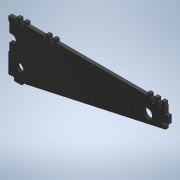
# Autodesk Inventor part: 10_ramie
Saved by Autodesk Inventor 2020.2 (Build 242310000, 310)
## iProperties
Created: 2017-10-07
Part Number: 10_ramie
Material: Ogólny
Document SubType Name: Modeling
Designer: Haras2
Density: 1 g/cm^3
Appearance: Gładki - czarny
Mass: 330.705 g
Surface Area: 962.933 cm^2
Volume: 330.705 cm^3
Author: Haras2
Autodesk Inventor part; units mm, degrees
ref_plane "YZ Plane" through (0, 0, 0) normal (1, 0, 0) x (0, 1, 0)
ref_plane "XZ Plane" through (0, 0, 0) normal (0, 1, 0) x (-1, 0, 0)
ref_plane "XY Plane" through (0, 0, 0) normal (0, 0, 1) x (1, 0, 0)
sketch "Szkic1" plane through (0, 0, 0) normal (0, 1, 0) x (-1, 0, 0)
  line L0 (0, 0) -> (0, -12)
  line L1 (0, -12) -> (-3, -15)
  line L2 (0, -137) -> (-15.5, -137)
  line L3 (-15.5, -137) -> (-15.5, -145)
  line L4 (-15.5, -145) -> (-35.5, -145)
  line L5 (-35.5, -145) -> (-35.5, -137)
  line L6 (-35.5, -137) -> (-47.5, -137)
  line L7 (-47.5, -137) -> (-421.5, -55)
  line L8 (-421.5, -55) -> (-421.5, -39.5)
  line L9 (-421.5, -39.5) -> (-429.5, -39.5)
  line L10 (-429.5, -39.5) -> (-429.5, -19.5)
  line L11 (-429.5, -19.5) -> (-421.5, -19.5)
  line L12 (-421.5, -19.5) -> (-421.5, 0)
  line L13 (-421.5, 0) -> (-419.5, 0)
  line L14 (-419.5, 0) -> (-419.5, 8)
  line L15 (-419.5, 8) -> (-411.5, 8)
  line L16 (-411.5, 8) -> (-411.5, 0)
  line L17 (-411.5, 0) -> (-400.5, 0)
  line L18 (-400.5, 0) -> (-400.5, 8)
  line L19 (-400.5, 8) -> (-392.5, 8)
  line L20 (-392.5, 8) -> (-392.5, 0)
  line L21 (-392.5, 0) -> (-381.5, 0)
  line L22 (-381.5, 0) -> (-381.5, 8)
  line L23 (-381.5, 8) -> (-373.5, 8)
  line L24 (-373.5, 8) -> (-373.5, 0)
  line L25 (-373.5, 0) -> (-128.5, 0)
  line L26 (-128.5, 0) -> (-128.5, 8)
  line L27 (-128.5, 8) -> (-120.5, 8)
  line L28 (-120.5, 8) -> (-120.5, 0)
  line L29 (-120.5, 0) -> (-110, 0)
  line L30 (-110, 0) -> (-110, 8)
  line L31 (-110, 8) -> (-102, 8)
  line L32 (-102, 8) -> (-102, 0)
  line L33 (-102, 0) -> (-50, 0)
  line L34 (-50, 0) -> (-50, 8)
  line L35 (-50, 8) -> (-42, 8)
  line L36 (-42, 8) -> (-42, 0)
  line L37 (-42, 0) -> (-31.5, 0)
  line L38 (-31.5, 0) -> (-31.5, 8)
  line L39 (-31.5, 8) -> (-23.5, 8)
  line L40 (-23.5, 8) -> (-23.5, 0)
  line L41 (-23.5, 0) -> (0, 0)
  line L42 (0, -137) -> (0, -84)
  line L43 (0, -84) -> (-3, -81)
  line L44 (-3, -49.75) -> (-9.75, -49.75) construction
  line L45 (-3, -60) -> (-9.75, -60)
  line L46 (-9.75, -39.5) -> (-3, -39.5)
  arc A0 (-9.75, -39.5) -> (-9.75, -60) centre (-9.75, -49.75) ccw
  line L47 (-3, -81) -> (-3, -60)
  line L48 (-3, -39.5) -> (-3, -15)
  line L49 (-385.25, -7) -> (-384, -7)
  line L50 (-384, -7) -> (-384, -4)
  line L51 (-384, -4) -> (-385.25, -4)
  line L52 (-385.25, -4) -> (-385.25, 0)
  line L53 (-385.25, 0) -> (-388.75, 0)
  line L54 (-388.75, 0) -> (-388.75, -4)
  line L55 (-388.75, -4) -> (-390, -4)
  line L56 (-390, -4) -> (-390, -7)
  line L57 (-390, -7) -> (-388.75, -7)
  line L58 (-388.75, -7) -> (-388.75, -12)
  line L59 (-388.75, -12) -> (-385.25, -12)
  line L60 (-385.25, -12) -> (-385.25, -7)
  line L61 (-387, 0) -> (-387, -12) construction
  line L62 (-404.25, -7) -> (-403, -7)
  line L63 (-403, -7) -> (-403, -4)
  line L64 (-403, -4) -> (-404.25, -4)
  line L65 (-404.25, -4) -> (-404.25, 0)
  line L66 (-404.25, 0) -> (-407.75, 0)
  line L67 (-407.75, 0) -> (-407.75, -4)
  line L68 (-407.75, -4) -> (-409, -4)
  line L69 (-409, -4) -> (-409, -7)
  line L70 (-409, -7) -> (-407.75, -7)
  line L71 (-407.75, -7) -> (-407.75, -12)
  line L72 (-407.75, -12) -> (-404.25, -12)
  line L73 (-404.25, -12) -> (-404.25, -7)
  line L74 (-406, 0) -> (-406, -12) construction
  line L75 (-414.5, -43.5) -> (-414.5, -42.25)
  line L76 (-414.5, -42.25) -> (-417.5, -42.25)
  line L77 (-417.5, -42.25) -> (-417.5, -43.5)
  line L78 (-417.5, -43.5) -> (-421.5, -43.5)
  line L79 (-421.5, -43.5) -> (-421.5, -47)
  line L80 (-421.5, -47) -> (-417.5, -47)
  line L81 (-417.5, -47) -> (-417.5, -48.25)
  line L82 (-417.5, -48.25) -> (-414.5, -48.25)
  line L83 (-414.5, -48.25) -> (-414.5, -47)
  line L84 (-414.5, -47) -> (-409.5, -47)
  line L85 (-409.5, -47) -> (-409.5, -43.5)
  line L86 (-409.5, -43.5) -> (-414.5, -43.5)
  line L87 (-421.5, -45.25) -> (-409.5, -45.25) construction
  line L88 (-113.5, -7) -> (-112.25, -7)
  line L89 (-112.25, -7) -> (-112.25, -4)
  line L90 (-112.25, -4) -> (-113.5, -4)
  line L91 (-113.5, -4) -> (-113.5, 0)
  line L92 (-113.5, 0) -> (-117, 0)
  line L93 (-117, 0) -> (-117, -4)
  line L94 (-117, -4) -> (-118.25, -4)
  line L95 (-118.25, -4) -> (-118.25, -7)
  line L96 (-118.25, -7) -> (-117, -7)
  line L97 (-117, -7) -> (-117, -12)
  line L98 (-117, -12) -> (-113.5, -12)
  line L99 (-113.5, -12) -> (-113.5, -7)
  line L100 (-115.25, 0) -> (-115.25, -12) construction
  line L101 (-95, -7) -> (-93.75, -7)
  line L102 (-93.75, -7) -> (-93.75, -4)
  line L103 (-93.75, -4) -> (-95, -4)
  line L104 (-95, -4) -> (-95, 0)
  line L105 (-95, 0) -> (-98.5, 0)
  line L106 (-98.5, 0) -> (-98.5, -4)
  line L107 (-98.5, -4) -> (-99.75, -4)
  line L108 (-99.75, -4) -> (-99.75, -7)
  line L109 (-99.75, -7) -> (-98.5, -7)
  line L110 (-98.5, -7) -> (-98.5, -12)
  line L111 (-98.5, -12) -> (-95, -12)
  line L112 (-95, -12) -> (-95, -7)
  line L113 (-96.75, 0) -> (-96.75, -12) construction
  line L114 (-35, -7) -> (-33.75, -7)
  line L115 (-33.75, -7) -> (-33.75, -4)
  line L116 (-33.75, -4) -> (-35, -4)
  line L117 (-35, -4) -> (-35, 0)
  line L118 (-35, 0) -> (-38.5, 0)
  line L119 (-38.5, 0) -> (-38.5, -4)
  line L120 (-38.5, -4) -> (-39.75, -4)
  line L121 (-39.75, -4) -> (-39.75, -7)
  line L122 (-39.75, -7) -> (-38.5, -7)
  line L123 (-38.5, -7) -> (-38.5, -12)
  line L124 (-38.5, -12) -> (-35, -12)
  line L125 (-35, -12) -> (-35, -7)
  line L126 (-36.75, 0) -> (-36.75, -12) construction
  line L127 (-16.5, -7) -> (-15.25, -7)
  line L128 (-15.25, -7) -> (-15.25, -4)
  line L129 (-15.25, -4) -> (-16.5, -4)
  line L130 (-16.5, -4) -> (-16.5, 0)
  line L131 (-16.5, 0) -> (-20, 0)
  line L132 (-20, 0) -> (-20, -4)
  line L133 (-20, -4) -> (-21.25, -4)
  line L134 (-21.25, -4) -> (-21.25, -7)
  line L135 (-21.25, -7) -> (-20, -7)
  line L136 (-20, -7) -> (-20, -12)
  line L137 (-20, -12) -> (-16.5, -12)
  line L138 (-16.5, -12) -> (-16.5, -7)
  line L139 (-18.25, 0) -> (-18.25, -12) construction
  line L140 (-11.75, -130) -> (-13, -130)
  line L141 (-13, -130) -> (-13, -133)
  line L142 (-13, -133) -> (-11.75, -133)
  line L143 (-11.75, -133) -> (-11.75, -137)
  line L144 (-11.75, -137) -> (-8.25, -137)
  line L145 (-8.25, -137) -> (-8.25, -133)
  line L146 (-8.25, -133) -> (-7, -133)
  line L147 (-7, -133) -> (-7, -130)
  line L148 (-7, -130) -> (-8.25, -130)
  line L149 (-8.25, -130) -> (-8.25, -125)
  line L150 (-8.25, -125) -> (-11.75, -125)
  line L151 (-11.75, -125) -> (-11.75, -130)
  line L152 (-10, -137) -> (-10, -125) construction
  line L153 (-42.75, -130) -> (-44, -130)
  line L154 (-44, -130) -> (-44, -133)
  line L155 (-44, -133) -> (-42.75, -133)
  line L156 (-42.75, -133) -> (-42.75, -137)
  line L157 (-42.75, -137) -> (-39.25, -137)
  line L158 (-39.25, -137) -> (-39.25, -133)
  line L159 (-39.25, -133) -> (-38, -133)
  line L160 (-38, -133) -> (-38, -130)
  line L161 (-38, -130) -> (-39.25, -130)
  line L162 (-39.25, -130) -> (-39.25, -125)
  line L163 (-39.25, -125) -> (-42.75, -125)
  line L164 (-42.75, -125) -> (-42.75, -130)
  line L165 (-41, -137) -> (-41, -125) construction
  point P0 (0, 0)
  point P1 (-30, -107)
  dimension "d5" = 137
  dimension "d6" = 45
  dimension "d7" = 12
  dimension "d8" = 53
  dimension "d9" = 23.5
  dimension "d10" = 8
  dimension "d11" = 10.5
  dimension "d12" = 8
  dimension "d13" = 10.5
  dimension "d14" = 11
  dimension "d15" = 11
  dimension "d16" = 421.5
  dimension "d17" = 55
  dimension "d18" = 8
  dimension "d19" = 20
  dimension "d20" = 19.5
  dimension "d21" = 102
  dimension "d22" = 373.5
  dimension "d23" = 20
  dimension "d24" = 15.5
  dimension "d25" = 8
  dimension "d26" = 47.5
  dimension "d27" = 3
  dimension "d28" = 20.5
  dimension "d29" = 39.5
  dimension "d30" = 17
  dimension "d31" = 4
  dimension "d32" = 3.5
  dimension "d33" = 3.5
  dimension "d34" = 3.75
  dimension "d35" = 3.75
  dimension "d38" = 30
  dimension "d39" = 30
  constraints: 99 end point, 30 point on line, 26 perpendicular, 16 horizontal, 8 collinear, 6 vertical, 2 parallel, 2 point on circle, 2 tangent, 1 centre point, 1 coincident
  measures "d5" distance between parallel lines of L2 L41
  measures "d6" angle of L0 L1
  measures "d7" distance of L0.start L0.end
  measures "d8" distance of L2.start L43.start
  measures "d9" distance between parallel lines of L0 L40
  measures "d10" distance of L38.end L39.end
  measures "d11" distance between parallel lines of L36 L38
  measures "d12" distance of L39.end L40.end
  measures "d13" distance between parallel lines of L28 L30
  measures "d14" distance between parallel lines of L20 L22
  measures "d15" distance between parallel lines of L16 L18
  measures "d16" distance between parallel lines of L0 L12
  measures "d17" distance from line of L13 L8.start
  measures "d18" distance of L11.start L12.start
  measures "d19" distance of L10.start L11.start
  measures "d20" distance between parallel lines of L13 L11
  measures "d21" distance between parallel lines of L0 L32
  measures "d22" distance between parallel lines of L0 L24
  measures "d23" distance of L3.end L4.end
  measures "d24" distance between parallel lines of L42 L3
  measures "d25" distance of L3.start L3.end
  measures "d26" distance from line of L6.end L42
  measures "d27" distance between parallel lines of L0 L48
  measures "d28" distance between parallel lines of L45 L46
  measures "d29" distance between parallel lines of L41 L46
  measures "d38" distance from line of L42 point (-30, -107)
  measures "d39" distance from line of L2 point (-30, -107)
extrude "Wyciągnięcie proste1" add sketch "Szkic1" along normal blind 8 contours L0 L1 L48 L46 A0 L45 L47 L43 L42 L2 L145 L146 L147 L148 L149 L150 L151 L140 L141 L142 L143 L3 L4 L5 L6 L158 L159 L160 L161 L162 L163 L164 L153 L154 L155 L156 L7 L8 L80 L81 L82 L83 L84 L85 L86 L75 L76 L77 L78 L9 L10 L11 L12 L13 L14 L15 L16 L17 L67 L68 L69 L70 L71 L72 L73 L62 L63 L64 L65 L18 L19 L20 L21 L54 L55 L56 L57 L58 L59 L60 L49 L50 L51 L52 L22 L23 L24 L25 L26 L27 L28 L29 L93 L94 L95 L96 L97 L98 L99 L88 L89 L90 L91 L30 L31 L32 L33 L106 L107 L108 L109 L110 L111 L112 L101 L102 L103 L104 L34 L35 L36 L37 L119 L120 L121 L122 L123 L124 L125 L114 L115 L116 L117 L38 L39 L40 L41 L132 L133 L134 L135 L136 L137 L138 L127 L128 L129 L130
sketch "Szkic2" plane through (0, 8, 0) normal (0, 1, 0) x (1, 0, 0)
  line L0 (0, 12) -> (0, 0) projected
  line L1 (50, 0) -> (95, 0) projected
  line L2 (0, 137) -> (0, 84) projected
  line L3 (8.25, 137) -> (0, 137) projected
  line L4 (128.5, 0) -> (373.5, 0) projected
  point P0 (30, 107)
  point P1 (131.5, 6)
  point P2 (131.5, 92.75)
  point P3 (80, 85)
  point P4 (80, 35)
  point P5 (223, 6)
  point P6 (230, 35)
  point P7 (223, 92)
  point P8 (373.5, 42)
  point P9 (338, 46.75)
  dimension "d56" = 80
  dimension "d57" = 35
  dimension "d58" = 30
  dimension "d59" = 30
  dimension "d63" = 92.75
  dimension "d64" = 6
  dimension "d65" = 131.5
  dimension "d66" = 92
  dimension "d67" = 223
  dimension "d69" = 46.75
  dimension "d70" = 42
  dimension "d71" = 373.5
  dimension "d72" = 338
  dimension "d95" = 50
  dimension "d96" = 150
  constraints: 3 vertical alignment, 2 horizontal alignment
  measures "d56" distance from line of L0 point (80, 35)
  measures "d57" distance from line of L1 point (80, 35)
  measures "d58" distance from line of L2 point (30, 107)
  measures "d59" distance from line of point (30, 107) L3
  measures "d63" distance from line of L1 point (131.5, 92.75)
  measures "d64" distance from line of L1 point (131.5, 6)
  measures "d65" distance from line of point (131.5, 6) L0
  measures "d66" distance from line of L4 point (223, 92)
  measures "d67" distance from line of L2 point (223, 92)
  measures "d69" distance from line of L4 point (338, 46.75)
  measures "d70" distance from line of L4 point (373.5, 42)
  measures "d71" distance from line of L0 point (373.5, 42)
  measures "d72" distance from line of point (338, 46.75) L0
  measures "d95" distance of point (80, 85) point (80, 35)
  measures "d96" distance of point (230, 35) point (80, 35)
hole "Otwór1" at (30, 8, -107) at (131.5, 8, -6) at (131.5, 8, -92.75) at (80, 8, -85) at (80, 8, -35) at (223, 8, -6) at (230, 8, -35) at (223, 8, -92) at (373.5, 8, -42) at (338, 8, -46.75) direction (0, -1, 0) diameter 3.5 end through all
sketch "Szkic3" plane through (0, 8, 0) normal (0, 1, 0) x (1, 0, 0)
  circle A0 centre (30, 107) radius 1.75 projected
  point P0 (0, 0)
  constraints: 1 coincident
hole "Otwór2" at (30, 8, -107) direction (0, -1, 0) diameter 20 end through all
sketch "Szkic4" plane through (0, 8, 0) normal (0, 1, 0) x (1, 0, 0)
  circle A0 centre (373.5, 42) radius 1.75 projected
  point P0 (0, 0)
  constraints: 1 coincident
hole "Otwór3" at (373.5, 8, -42) direction (0, -1, 0) diameter 25 end through all
fillet "Zaokrąglenie1" radius 2 8 edges at (0, 4, -137) (0, 4, -84) (3, 4, -81) (3, 4, -60) (3, 4, -39.5) (3, 4, -15) (0, 4, -12) (0, 4, 0)
sketch "Sketch5" plane through (0, 0, 0) normal (0, -1, 0) x (1, 0, 0)
  circle A0 centre (387, -5.5) radius 2.5
  line L0 (388.75, 0) -> (388.75, -4) projected
  line L1 (385.25, -7) -> (384, -7) projected
  circle A1 centre (115.25, -5.5) radius 2.5
  line L2 (117, 0) -> (117, -4) projected
  circle A2 centre (41, -131.5) radius 2.5
  line L3 (42.75, -125) -> (42.75, -130) projected
  line L4 (38, -130) -> (39.25, -130) projected
  point P0 (0, 0)
  dimension "d97" = 1.75
  dimension "d98" = 1.5
  dimension "d99" = 5
  dimension "d100" = 1.75
  dimension "d101" = 1.75
  dimension "d102" = 1.5
  constraints: 3 centre point, 2 equal radius
  measures "d97" distance from line of L0 A0.centre
  measures "d98" distance from line of L1 A0.centre
  measures "d99" diameter of A0
  measures "d100" distance from line of L2 A1.centre
  measures "d101" distance from line of A2.centre L3
  measures "d102" distance from line of L4 A2.centre
sketch "Block1" plane through (0, 0, 0) normal (0, 0, 1) x (1, 0, 0)
  line L0 (-406.7655, -141.7615) -> (-405.5155, -141.7615)
  line L1 (-405.5155, -141.7615) -> (-405.5155, -138.7615)
  line L2 (-405.5155, -138.7615) -> (-406.7655, -138.7615)
  line L3 (-406.7655, -138.7615) -> (-406.7655, -134.7615)
  line L4 (-406.7655, -134.7615) -> (-410.2655, -134.7615)
  line L5 (-410.2655, -134.7615) -> (-410.2655, -138.7615)
  line L6 (-410.2655, -138.7615) -> (-411.5155, -138.7615)
  line L7 (-411.5155, -138.7615) -> (-411.5155, -141.7615)
  line L8 (-411.5155, -141.7615) -> (-410.2655, -141.7615)
  line L9 (-410.2655, -141.7615) -> (-410.2655, -146.7615)
  line L10 (-410.2655, -146.7615) -> (-406.7655, -146.7615)
  line L11 (-406.7655, -146.7615) -> (-406.7655, -141.7615)
  line L12 (-408.5155, -134.7615) -> (-408.5155, -146.7615) construction
  dimension "d0" = 4
  dimension "d1" = 3
  dimension "d2" = 5
  dimension "d3" = 3.5
  dimension "d4" = 6
  constraints: 26 end point, 5 collinear, 4 perpendicular, 3 parallel, 2 midpoint, 1 coincident, 1 horizontal, 1 other
  measures "d0" distance of L4.end L5.end
  measures "d1" distance of L6.end L7.end
  measures "d2" distance of L8.end L9.end
  measures "d3" distance of L3.end L4.end
  measures "d4" distance between parallel lines of L1 L7
